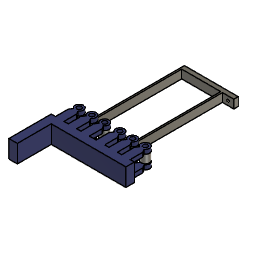
Modelo Analisis Estructural (Autodesk Fusion 360 design; units mm, degrees)
Autodesk Fusion 360 part; units mm, degrees
note: some values were not read from the file. Set by a fixed rule: which sketch regions a step uses.
sketch "Boceto1" plane through (0, 0, 0) normal (0, 0, 1) x (1, 0, 0)
  circle A0 centre (0, 0) radius 2.65
  circle A1 centre (48, 0) radius 2.65
  circle A2 centre (0, 0) radius 5
  circle A3 centre (48, 0) radius 5
  line L0 (-25, -8) -> (73, -8)
  line L1 (73, -8) -> (73, -18)
  line L2 (73, -18) -> (-25, -18)
  line L3 (-25, -18) -> (-25, -8)
  line L4 (0, 0) -> (-5, -8)
  line L5 (0, 0) -> (5, -8)
  line L6 (48, 0) -> (43, -8)
  line L7 (48, 0) -> (53, -8)
  line L8 (0, 0) -> (48, 0) construction
  circle A4 centre (15, 0) radius 2.65
  circle A5 centre (15, 0) radius 5
  circle A6 centre (33, 0) radius 2.65
  circle A7 centre (33, 0) radius 5
  circle A8 centre (63, 0) radius 2.65
  circle A9 centre (63, 0) radius 5
  circle A10 centre (-15, 0) radius 5
  circle A11 centre (-15, 0) radius 2.65
  line L9 (-15, 5) -> (63, 5) construction
  line L10 (-15, 2.65) -> (63, 2.65) construction
  line L11 (-15, 0) -> (0, 0) construction
  line L12 (63, 0) -> (48, 0) construction
  line L13 (-15, 0) -> (-20, -8)
  line L14 (-15, 0) -> (-10, -8)
  line L15 (15, 0) -> (10, -8)
  line L16 (15, 0) -> (20, -8)
  line L17 (33, 0) -> (28, -8)
  line L18 (33, 0) -> (38, -8)
  line L19 (63, 0) -> (58, -8)
  line L20 (63, 0) -> (68, -8)
  dimension "d1" = 5.3
  dimension "d6" = 10
  dimension "d8" = 8
  dimension "d11" = 48
  dimension "d16" = 15
  dimension "d17" = 15
  dimension "d18" = 15
  dimension "d19" = 15
  dimension "d20" = 98
  dimension "d21" = 10
  dimension "d22" = 25
  constraint coincident A0.centre A2.centre
  constraint concentric A0 A2
  constraint concentric A1 A3
  constraint horizontal L0
  constraint vertical L1
  constraint horizontal L2
  constraint vertical L3
  constraint coincident L0 L4.end
  constraint coincident L0 L5.end
  constraint coincident A1.centre A3.centre
  constraint coincident L0 L6.end
  constraint coincident L0 L7.end
  constraint parallel L5 L7
  constraint equal L4 L5
  constraint equal L6 L7
  constraint horizontal L8
  constraint coincident L8 A4.centre
  constraint concentric A4 A5
  constraint coincident L8 A6.centre
  constraint concentric A6 A7
  constraint concentric A8 A9
  constraint concentric A10 A11
  constraint coincident A10 L9.start
  constraint horizontal L9
  constraint coincident A11 L10.start
  constraint horizontal L10
  constraint tangent A0 L10
  constraint tangent A2 L9
  constraint tangent A5 L9
  constraint tangent A4 L10
  constraint tangent A6 L10
  constraint tangent A7 L9
  constraint tangent A3 L9
  constraint tangent A1 L10
  constraint tangent A8 L10
  constraint tangent A9 L9
  constraint tangent A10 L9
  constraint tangent A11 L10
  constraint coincident A10.centre A11.centre
  constraint coincident A8.centre A9.centre
  constraint horizontal L12
  constraint horizontal L11
  constraint coincident A8 L10.end
  constraint coincident A9 L9.end
  constraint coincident L0 L13.end
  constraint coincident L0 L14.end
  constraint coincident A4.centre A5.centre
  constraint coincident L0 L15.end
  constraint coincident L0 L16.end
  constraint parallel L14 L16
  constraint coincident A6.centre A7.centre
  constraint coincident L0 L17.end
  constraint parallel L15 L17
  constraint coincident L0 L18.end
  constraint parallel L16 L18
  constraint coincident L0 L19.end
  constraint parallel L17 L19
  constraint coincident L0 L20.end
  constraint parallel L18 L20
  constraint equal L13 L14
  constraint equal L4 L14
  constraint equal L15 L16
  measures "d1" diameter of A0
  measures "d6" diameter of A2
  measures "d8" distance of A0.centre L0
  measures "d11" distance of A1.centre A0.centre
  measures "d16" distance of A0.centre A10.centre
  measures "d17" distance of A0.centre A4.centre
  measures "d18" distance of A1.centre A6.centre
  measures "d19" distance of A1.centre A8.centre
  measures "d20" distance of L1.end L2.end
  measures "d21" distance of L0.start L2.end
  measures "d22" distance of A0.centre L3
extrude "Extruir1" add sketch "Boceto1" along normal blind 21 contours A0 A2 L4 L5 | A0 A2 L4 L5 | A2 L0 L4 L5 | L0 L1 L2 L3 | L0 A10 L13 L14 | L0 A5 L15 L16 | A10 A11 L13 L14 | A10 A11 L13 L14 | A4 A5 L15 L16 | A4 A5 L15 L16 | L0 A7 L17 L18 | A6 A7 L17 L18 | A6 A7 L17 L18 | A3 L0 L6 L7 | A1 A3 L6 L7 | A1 A3 L6 L7 | L0 A9 L19 L20 | A8 A9 L19 L20 | A8 A9 L19 L20 makes body 1
sketch "Boceto2" plane through (-25, 0, 0) normal (-1, 0, 0) x (0, -1, 0)
  line L0 (8, 0) -> (18, 0)
  line L1 (18, 0) -> (18, 21)
  line L2 (18, 21) -> (8, 21)
  line L3 (8, 21) -> (8, 0)
  line L4 (8, 10.5) -> (-7.6781, 10.5)
  line L5 (-7.6781, 10.5) -> (-7.6781, 5)
  line L6 (-7.6781, 5) -> (8, 5)
  line L7 (8, 5) -> (8, 10.5)
  line L8 (8, 10.5) -> (-7.9551, 10.5)
  line L9 (-7.9551, 10.5) -> (-7.9551, 16)
  line L10 (-7.9551, 16) -> (8, 16)
  line L11 (8, 16) -> (8, 10.5)
  dimension "d23" = 11
  constraint horizontal L4
  constraint vertical L5
  constraint horizontal L6
  constraint vertical L7
  constraint midpoint L3 L4.start
  constraint horizontal L8
  constraint vertical L9
  constraint horizontal L10
  constraint vertical L11
  constraint equal L7 L11
  measures "d23" distance of L6 L10
extrude "Extruir2" cut sketch "Boceto2" against normal through all contours L3 L4 L5 L6 L7 L8 | L3 L4 L8 L9 L10 L11 bodies 1
extrude "Extruir3" add sketch "Boceto1" along normal blind 1 contours A3 L0 L6 L7 bodies 1
sketch "Boceto4" plane through (0, 0, 0) normal (0, 0, -1) x (1, 0, 0)
  circle A0 centre (48, 0) radius 3
  circle A1 centre (0, 0) radius 3
  circle A2 centre (63, 0) radius 3
  circle A3 centre (15, 0) radius 3
  circle A4 centre (33, 0) radius 3
  arc A5 (-17.65, 4.24) -> (-12.35, 4.24) centre (-15, 0) ccw
  line L0 (-12.35, 4.24) -> (-10, 8)
  line L1 (-10, 8) -> (-5, 8)
  line L2 (-5, 8) -> (-2.65, 4.24)
  arc A6 (-2.65, 4.24) -> (2.65, 4.24) centre (0, 0) ccw
  line L3 (2.65, 4.24) -> (5, 8)
  line L4 (5, 8) -> (10, 8)
  line L5 (10, 8) -> (12.35, 4.24)
  arc A7 (12.35, 4.24) -> (17.65, 4.24) centre (15, 0) ccw
  line L6 (17.65, 4.24) -> (20, 8)
  line L7 (20, 8) -> (28, 8)
  line L8 (28, 8) -> (30.35, 4.24)
  arc A8 (30.35, 4.24) -> (35.65, 4.24) centre (33, 0) ccw
  line L9 (35.65, 4.24) -> (38, 8)
  line L10 (38, 8) -> (43, 8)
  line L11 (43, 8) -> (45.35, 4.24)
  arc A9 (45.35, 4.24) -> (50.65, 4.24) centre (48, 0) ccw
  line L12 (50.65, 4.24) -> (53, 8)
  line L13 (53, 8) -> (58, 8)
  line L14 (58, 8) -> (60.35, 4.24)
  arc A10 (60.35, 4.24) -> (65.65, 4.24) centre (63, 0) ccw
  line L15 (65.65, 4.24) -> (68, 8)
  line L16 (68, 8) -> (73, 8)
  line L17 (73, 8) -> (73, 18)
  line L18 (73, 18) -> (-25, 18)
  line L19 (-25, 18) -> (-25, 8)
  line L20 (-25, 8) -> (-20, 8)
  line L21 (-20, 8) -> (-17.65, 4.24)
  circle A11 centre (-15, 0) radius 3
  circle A12 centre (48, 13) radius 4
  circle A13 centre (0, 13) radius 4
  line L22 (48, 0) -> (48, 13) construction
  line L23 (0, 0) -> (0, 13) construction
  line L24 (48, 13) -> (0, 13) construction
  dimension "d36" = 5.2
  dimension "d37" = 8
  dimension "d38" = 8
  constraint coincident A0.centre A9.centre
  constraint coincident A12.centre L22.end
  constraint coincident A1.centre A6.centre
  constraint coincident A13.centre L23.end
  constraint vertical L23
  constraint vertical L22
  constraint horizontal L24
  measures "d37" diameter of A12
  measures "d38" diameter of A13
extrude "Extruir5" [suppressed]
sketch "Boceto5" plane through (0, 0, 0) normal (0, 0, -1) x (1, 0, 0)
  circle A0 centre (48, 0) radius 2.65
  circle A1 centre (0, 0) radius 2.65
  circle A2 centre (63, 0) radius 2.65
  circle A3 centre (15, 0) radius 2.65
  circle A4 centre (33, 0) radius 2.65
  arc A5 (-17.65, 4.24) -> (-12.35, 4.24) centre (-15, 0) ccw
  line L0 (-12.35, 4.24) -> (-10, 8)
  line L1 (-10, 8) -> (-5, 8)
  line L2 (-5, 8) -> (-2.65, 4.24)
  arc A6 (-2.65, 4.24) -> (2.65, 4.24) centre (0, 0) ccw
  line L3 (2.65, 4.24) -> (5, 8)
  line L4 (5, 8) -> (10, 8)
  line L5 (10, 8) -> (12.35, 4.24)
  arc A7 (12.35, 4.24) -> (17.65, 4.24) centre (15, 0) ccw
  line L6 (17.65, 4.24) -> (20, 8)
  line L7 (20, 8) -> (28, 8)
  line L8 (28, 8) -> (30.35, 4.24)
  arc A8 (30.35, 4.24) -> (35.65, 4.24) centre (33, 0) ccw
  line L9 (35.65, 4.24) -> (38, 8)
  line L10 (38, 8) -> (43, 8)
  line L11 (43, 8) -> (45.35, 4.24)
  arc A9 (45.35, 4.24) -> (50.65, 4.24) centre (48, 0) ccw
  line L12 (50.65, 4.24) -> (53, 8)
  line L13 (53, 8) -> (58, 8)
  line L14 (58, 8) -> (60.35, 4.24)
  arc A10 (60.35, 4.24) -> (65.65, 4.24) centre (63, 0) ccw
  line L15 (65.65, 4.24) -> (68, 8)
  line L16 (68, 8) -> (73, 8)
  line L17 (73, 8) -> (73, 18)
  line L18 (73, 18) -> (-25, 18)
  line L19 (-25, 18) -> (-25, 8)
  line L20 (-25, 8) -> (-20, 8)
  line L21 (-20, 8) -> (-17.65, 4.24)
  circle A11 centre (-15, 0) radius 2.65
  line L22 (73, 18) -> (-25, 18)
  line L23 (-25, 18) -> (-25, 8)
  line L24 (-25, 8) -> (73, 8)
  line L25 (73, 8) -> (73, 18)
  constraint horizontal L22
  constraint vertical L23
  constraint horizontal L24
  constraint vertical L25
  constraint coincident L19.end L20.start
  constraint coincident L17.end L18.start
extrude "Extruir6" add sketch "Boceto5" along normal blind 50 separate body contours L1 L4 L7 L10 L13 L16 L17 L18 L19 L20 L22 L23 L24 L25 makes body 2
pattern_linear "Patrón R2" count 3 spacing 80 along (0, 0, -1) of bodies 1 makes body 3 at (40.3333, -18, -73) makes body 4 at (40.3333, -18, -153)
pattern_linear "Patrón R3" count 2 spacing 80 along (0, 0, -1) of bodies 2 makes body 5
sketch "Boceto6" plane through (0, 0, -160) normal (0, 0, -1) x (1, 0, 0)
  circle A0 centre (48, 13) radius 4
  circle A1 centre (0, 13) radius 4
  circle A2 centre (48, 0) radius 3
  circle A3 centre (0, 0) radius 3
  circle A4 centre (63, 0) radius 3
  circle A5 centre (15, 0) radius 3
  circle A6 centre (33, 0) radius 3
  arc A7 (-17.65, 4.24) -> (-12.35, 4.24) centre (-15, 0) ccw
  line L0 (-12.35, 4.24) -> (-10, 8)
  line L1 (-10, 8) -> (-5, 8)
  line L2 (-5, 8) -> (-2.65, 4.24)
  arc A8 (-2.65, 4.24) -> (2.65, 4.24) centre (0, 0) ccw
  line L3 (2.65, 4.24) -> (5, 8)
  line L4 (5, 8) -> (10, 8)
  line L5 (10, 8) -> (12.35, 4.24)
  arc A9 (12.35, 4.24) -> (17.65, 4.24) centre (15, 0) ccw
  line L6 (17.65, 4.24) -> (20, 8)
  line L7 (20, 8) -> (28, 8)
  line L8 (28, 8) -> (30.35, 4.24)
  arc A10 (30.35, 4.24) -> (35.65, 4.24) centre (33, 0) ccw
  line L9 (35.65, 4.24) -> (38, 8)
  line L10 (38, 8) -> (43, 8)
  line L11 (43, 8) -> (45.35, 4.24)
  arc A11 (45.35, 4.24) -> (50.65, 4.24) centre (48, 0) ccw
  line L12 (50.65, 4.24) -> (53, 8)
  line L13 (53, 8) -> (58, 8)
  line L14 (58, 8) -> (60.35, 4.24)
  arc A12 (60.35, 4.24) -> (65.65, 4.24) centre (63, 0) ccw
  line L15 (65.65, 4.24) -> (68, 8)
  line L16 (68, 8) -> (73, 8)
  line L17 (73, 8) -> (73, 18)
  line L18 (73, 18) -> (-25, 18)
  line L19 (-25, 18) -> (-25, 8)
  line L20 (-25, 8) -> (-20, 8)
  line L21 (-20, 8) -> (-17.65, 4.24)
  circle A13 centre (-15, 0) radius 3
  circle A14 centre (63, 0) radius 3
  circle A15 centre (48, 0) radius 3
  circle A16 centre (33, 0) radius 3
  circle A17 centre (15, 0) radius 3
  circle A18 centre (0, 0) radius 3
  circle A19 centre (-15, 0) radius 3
  circle A20 centre (0, 13) radius 4
  circle A21 centre (48, 13) radius 4
extrude "Extruir7" [suppressed]
sketch "Boceto7" plane through (0, 0, 16) normal (0, 0, -1) x (1, 0, 0)
  arc A0 (60.35, 4.24) -> (65.65, 4.24) centre (63, 0) ccw
  circle A1 centre (63, 0) radius 2.65
  circle A2 centre (48, 0) radius 2.65
  arc A3 (45.35, 4.24) -> (50.65, 4.24) centre (48, 0) ccw
  arc A4 (30.35, 4.24) -> (35.65, 4.24) centre (33, 0) ccw
  circle A5 centre (33, 0) radius 2.65
  arc A6 (12.35, 4.24) -> (17.65, 4.24) centre (15, 0) ccw
  circle A7 centre (15, 0) radius 2.65
  arc A8 (-2.65, 4.24) -> (2.65, 4.24) centre (0, 0) ccw
  circle A9 centre (0, 0) radius 2.65
  arc A10 (-17.65, 4.24) -> (-12.35, 4.24) centre (-15, 0) ccw
  circle A11 centre (-15, 0) radius 2.65
  arc A12 (60.456, 4.0704) -> (60.4559, 4.0703) centre (63, 0) ccw
  arc A13 (60.4559, 4.0703) -> (60.456, 4.0704) centre (57.912, 8.1408) ccw
  circle A14 centre (48, 0) radius 4.8
  circle A15 centre (33, 0) radius 4.8
  circle A16 centre (15, 0) radius 4.8
  circle A17 centre (0, 0) radius 4.8
  circle A18 centre (-15, 0) radius 4.8
  line L0 (63, 0) -> (-15, 0) construction
  line L1 (58.4404, -1.5) -> (52.5596, -1.5)
  line L2 (58.4404, 1.5) -> (52.5596, 1.5)
  line L3 (43.4404, -1.5) -> (37.5596, -1.5)
  line L4 (43.4404, 1.5) -> (37.5596, 1.5)
  line L5 (10.4404, -1.5) -> (4.5596, -1.5)
  line L6 (10.4404, 1.5) -> (4.5596, 1.5)
  line L7 (-4.5596, -1.5) -> (-10.4404, -1.5)
  line L8 (-4.5596, 1.5) -> (-10.4404, 1.5)
  line L9 (48, -4.8) -> (0, -4.8) construction
  line L10 (0, -4.8) -> (0, -104.8) construction
  line L11 (0, -104.8) -> (48, -104.8)
  line L12 (48, -104.8) -> (48, -4.8) construction
  line L13 (47, -104.8) -> (47, -4.6947)
  line L14 (49, -104.8) -> (49, -4.6947)
  line L15 (1, -104.8) -> (1, -4.6947)
  line L16 (-1, -104.8) -> (-1, -4.6947)
  line L17 (49, -104.8) -> (-1, -104.8)
  line L18 (-1, -104.8) -> (-1, -110)
  line L19 (-1, -110) -> (49, -110)
  line L20 (49, -110) -> (49, -104.8)
  line L21 (65.65, 4.24) -> (68, 8)
  line L22 (68, 8) -> (58, 8)
  line L23 (58, 8) -> (60.35, 4.24)
  line L24 (35.65, 4.24) -> (38, 8)
  line L25 (38, 8) -> (28, 8)
  line L26 (28, 8) -> (30.35, 4.24)
  line L27 (17.65, 4.24) -> (20, 8)
  line L28 (20, 8) -> (10, 8)
  line L29 (10, 8) -> (12.35, 4.24)
  line L30 (-12.35, 4.24) -> (-10, 8)
  line L31 (-10, 8) -> (-20, 8)
  line L32 (-20, 8) -> (-17.65, 4.24)
  line L33 (50.65, 4.24) -> (53, 8)
  line L34 (53, 8) -> (43, 8)
  line L35 (43, 8) -> (45.35, 4.24)
  line L36 (2.65, 4.24) -> (5, 8)
  line L37 (5, 8) -> (-5, 8)
  line L38 (-5, 8) -> (-2.65, 4.24)
  circle A19 centre (63, 0) radius 4.8
  dimension "d56" = 3
  dimension "d58" = 100
  dimension "d59" = 2
  dimension "d60" = 1
  dimension "d61" = 2
  dimension "d62" = 1
  dimension "d63" = 5.2
  constraint concentric A2 A14
  constraint equal A12 A14
  constraint equal A14 A15
  constraint equal A15 A16
  constraint equal A16 A17
  constraint equal A17 A18
  constraint coincident A0.centre A1.centre
  constraint coincident A10.centre A11.centre
  constraint coincident A12 L1.start
  constraint coincident A14 L1.end
  constraint horizontal L1
  constraint coincident A12 L2.start
  constraint coincident A14 L2.end
  constraint parallel L1 L2
  constraint coincident A14 L3.start
  constraint coincident A15 L3.end
  constraint parallel L2 L3
  constraint coincident A14 L4.start
  constraint coincident A15 L4.end
  constraint horizontal L4
  constraint coincident A16 L5.start
  constraint coincident A17 L5.end
  constraint horizontal L5
  constraint coincident A16 L6.start
  constraint coincident A17 L6.end
  constraint parallel L5 L6
  constraint coincident A17 L7.start
  constraint coincident A18 L7.end
  constraint parallel L6 L7
  constraint coincident A17 L8.start
  constraint coincident A18 L8.end
  constraint parallel L7 L8
  constraint symmetric L0 L1 L2
  constraint symmetric L0 L3 L4
  constraint symmetric L0 L5 L6
  constraint symmetric L0 L7 L8
  constraint collinear L1 L3
  constraint collinear L3 L5
  constraint collinear L5 L7
  constraint horizontal L9
  constraint vertical L10
  constraint horizontal L11
  constraint vertical L12
  constraint coincident A14 L9.start
  constraint coincident A2.centre L12
  constraint coincident A8.centre L10
  constraint perpendicular L11 L13
  constraint parallel L12 L14
  constraint vertical L15
  constraint parallel L10 L16
  constraint coincident A14 L13.end
  constraint coincident A14 L14.end
  constraint coincident A17 L15.end
  constraint coincident A17 L16.end
  constraint coincident L11 L15.start
  constraint coincident L11 L13.start
  constraint horizontal L17
  constraint vertical L18
  constraint horizontal L19
  constraint vertical L20
  constraint collinear L11 L17
  constraint concentric A0 A12
  constraint tangent A12 A13
  constraint concentric A12 A19
  constraint equal A15 A19
  measures "d56" distance of L1 L2
  measures "d58" distance of L9.start L11.end
  measures "d59" distance of L13 L14
  measures "d60" distance of L12 L13
  measures "d61" distance of L15 L16
  measures "d62" distance of L10 L15
  measures "d63" distance of L14.start L19.end
extrude "Extruir8" add sketch "Boceto7" along normal blind 10 separate body contours A0 A12 L1 L2 A19 | A0 A3 L1 L2 | A12 A19 | A3 A14 L1 L2 | A14 | A3 L11 L13 L14 L17 | A3 A14 L13 L14 | A3 A14 L3 L4 | L11 L17 L18 L19 L20 | A3 A4 L3 L4 | A4 A15 L3 L4 | A8 L11 L15 L16 L17 | A15 | A8 A17 L15 L16 | A8 A17 L5 L6 | A6 A8 L5 L6 | A17 | A8 A10 L7 L8 | A8 A17 L7 L8 | A6 A16 L5 L6 | A10 A18 L7 L8 | A16 | A18 makes body 6
sketch "Boceto8" plane through (0, 110, 0) normal (0, 1, 0) x (-1, 0, 0)
  line L0 (1, 16) -> (-49, 16)
  line L1 (-49, 16) -> (-49, 6)
  line L2 (-49, 6) -> (1, 6)
  line L3 (1, 6) -> (1, 16)
  line L4 (-49, 11) -> (1, 11) construction
  circle A0 centre (-39, 11) radius 2.6
  circle A1 centre (-9, 11) radius 2.6
  dimension "d66" = 5.2
  dimension "d67" = 5.2
  dimension "d68" = 10
  dimension "d69" = 30
  constraint midpoint L1 L4.start
  constraint midpoint L3 L4.end
  constraint coincident L4 A0.centre
  constraint coincident L4 A1.centre
  measures "d66" diameter of A0
  measures "d67" diameter of A1
  measures "d68" distance of L1 A0.centre
  measures "d69" distance of A0.centre A1.centre
extrude "Extruir9" [suppressed]
extrude "Extruir10" add sketch "Boceto7" along normal blind 20 separate body contours A14 | A3 L11 L13 L14 L17 | A3 A14 L13 L14 | L11 L17 L18 L19 L20 | A8 L11 L15 L16 L17 | A8 A17 L15 L16 | A17 makes body 7
sketch "Boceto9" plane through (0, 59.8, 0) normal (0, 1, 0) x (-1, 0, 0)
  line L0 (1, 25.5) -> (-49, 25.5)
  line L1 (-49, 25.5) -> (-49, 5.5)
  line L2 (-49, 5.5) -> (1, 5.5)
  line L3 (1, 5.5) -> (1, 25.5)
  line L4 (-49, 15.5) -> (1, 15.5) construction
  circle A0 centre (-39, 15.5) radius 2.5
  circle A1 centre (-9, 15.5) radius 2.5
  dimension "d75" = 5.2
  dimension "d76" = 5.2
  dimension "d77" = 10
  dimension "d78" = 30
  constraint midpoint L1 L4.start
  constraint midpoint L3 L4.end
  constraint coincident L4 A0.centre
  constraint coincident L4 A1.centre
  measures "d77" distance of L1 A0.centre
  measures "d78" distance of A0.centre A1.centre
extrude "Extruir11" [suppressed]
pattern_linear "Patrón R4" count 3 spacing 80 along (0, 0, -1) of bodies 7 makes body 8 at (-1, 71.4997, -70.6667) makes body 9 at (-1, 71.4997, -150.6667)
sketch "Boceto10" plane through (49, 0, 0) normal (1, 0, 0) x (0, 1, 0)
  line L0 (59.8, 25.5) -> (4.6947, 25.5)
  line L1 (4.6947, 25.5) -> (4.6947, 5.5)
  line L2 (4.6947, 5.5) -> (59.8, 5.5)
  line L3 (59.8, 5.5) -> (59.8, 25.5)
  line L4 (59.8, 25.5) -> (55.2846, 25.5)
  line L5 (55.2846, 25.5) -> (55.2846, 5.5)
  line L6 (55.2846, 5.5) -> (59.8, 5.5)
  line L7 (59.8, 5.5) -> (59.8, 25.5)
  constraint horizontal L4
  constraint vertical L5
  constraint horizontal L6
  constraint vertical L7
  constraint coincident L2 L5.end
  constraint coincident L0.start L3.end
extrude "Extruir12" [suppressed]
hole "Agujero1" [suppressed]
sketch "Boceto11" plane through (49, 0, 0) normal (1, 0, 0) x (0, 1, 0)
  line L0 (110, 16) -> (4.6947, 16)
  line L1 (4.6947, 16) -> (4.6947, 6)
  line L2 (4.6947, 6) -> (110, 6)
  line L3 (110, 6) -> (110, 16)
  line L4 (55, 75) -> (60, 75)
  line L5 (110, 16) -> (104.8, 16)
  line L6 (104.8, 16) -> (104.8, -68.7489)
  line L7 (104.8, -68.7489) -> (110, -68.7489)
  line L8 (110, -68.7489) -> (110, 16)
  dimension "d100" = 5.2
  constraint horizontal L4
  constraint horizontal L5
  constraint vertical L6
  constraint horizontal L7
  constraint vertical L8
  constraint coincident L0.start L3.end
  measures "d100" distance of L0.start L5.end
extrude "Extruir13" add sketch "Boceto11" along normal blind 10 contours L0 L2 L3 L5 L6 L8 bodies 6
sketch "Boceto13" plane through (0, 110, 0) normal (0, 1, 0) x (-1, 0, 0)
  line L0 (1, 16) -> (-59, 16)
  line L1 (-59, 16) -> (-59, 6)
  line L2 (-59, 6) -> (1, 6)
  line L3 (1, 6) -> (1, 16)
  line L4 (-59, 16) -> (-59, 11)
  line L5 (-59, 11) -> (1, 11)
  line L6 (-49, 6) -> (-49, 16)
  line L7 (-49, 16) -> (-49, 6)
  point P0 (-55.75, 11)
  dimension "d122" = 6.75
  constraint coincident L0.end L1.start
  constraint midpoint L1 L4.end
  constraint midpoint L3 L5.end
  constraint coincident L5 P0
  measures "d122" distance of P0 L7
hole "Agujero2" at (55.75, 110, 11) direction (0, -1, 0) diameter 3 depth 10 tip angle 180 bodies 6
sketch "Boceto12" plane through (0, -18, 0) normal (0, -1, 0) x (1, 0, 0)
  line L0 (-25, 0) -> (73, 0)
  line L1 (73, 0) -> (73, 21)
  line L2 (73, 21) -> (-25, 21)
  line L3 (-25, 21) -> (-25, 0)
  line L4 (-25, 21) -> (-24, 21)
  line L5 (-24, 21) -> (-24, 1)
  line L6 (-24, 1) -> (-25, 1)
  line L7 (-25, 1) -> (-25, 21)
  dimension "d106" = 1
  constraint horizontal L4
  constraint vertical L5
  constraint horizontal L6
  constraint vertical L7
  constraint coincident L2.end L3.start
  measures "d106" distance of L2.end L4.end
extrude "Extruir14" [suppressed]
moveface "MoveFace1" [suppressed]
extrude "Extruir15" add 1 faces at (59, 106.5333, 9.3333) along direction (1, 0, 0) blind 1 on bodies 6 bodies 6
extrude "Extruir16" add 1 faces at (60, 106.5333, 9.3333) along direction (1, 0, 0) blind 0.5 on bodies 6 bodies 6
extrude "Extruir17" add 1 faces at (60.5, 106.5333, 9.3333) along direction (1, 0, 0) blind 2 on bodies 6 bodies 6
extrude "Extruir18" add 1 faces at (40.3333, -18, 7) along direction (0, -1, 0) blind 15 on bodies 1 bodies 1
extrude "Extruir19" cut 1 faces at (61.3333, -8, 12.3333) along direction (0, -1, 0) blind 15 on bodies 1 bodies 1
sketch "Boceto14" plane through (0, -33, 0) normal (0, -1, 0) x (1, 0, 0)
  line L0 (-25, 0) -> (73, 0)
  line L1 (73, 0) -> (73, 21)
  line L2 (73, 21) -> (-25, 21)
  line L3 (-25, 21) -> (-25, 0)
  line L4 (-25, 21) -> (-15, 21)
  line L5 (-15, 21) -> (-15, 0)
  line L6 (-15, 0) -> (-25, 0)
  line L7 (-25, 0) -> (-25, 21)
  dimension "d123" = 10
  constraint horizontal L4
  constraint vertical L5
  constraint horizontal L6
  constraint vertical L7
  constraint coincident L2.end L3.start
  constraint coincident L0.start L3.end
  measures "d123" distance of L2.end L4.end
extrude "Extruir20" add sketch "Boceto14" along normal blind 40 contours L0 L2 L3 L4 L5 L6 L7 bodies 1
hidden bodies 2 3 4 5 7 8 9
equation "d2 = AnchoBase + 11 mm"
equation "d23 = AnchoBase + 1 mm"
equation "d38 = d37"
equation "d58 = altura_marco"
equation "d64 = AnchoBase"
equation "d67 = d66"
equation "altura_marco = 100 mm"
equation "AnchoBase = 10 mm"
equation "EspesorColumna = 2 mm"
equation "d122 = ( 13.5 / 2 ) * 1 mm"
named bodies: "Base Marco Plano", "Marco Plano"
